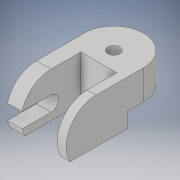
# Autodesk Inventor part: knuckle
Saved by Autodesk Inventor 2018 (Build 220112000, 112)
## iProperties
Created: 2017-10-01
Part Number: knuckle
Material: Generic
Document SubType Name: Modeling
Designer: Martin
Density: 1 g/cm^3
Appearance: Default
Author: Martin
Autodesk Inventor part; units mm, degrees
ref_plane "YZ Plane" through (0, 0, 0) normal (1, 0, 0) x (0, 1, 0)
ref_plane "XZ Plane" through (0, 0, 0) normal (0, 1, 0) x (-1, 0, 0)
ref_plane "XY Plane" through (0, 0, 0) normal (0, 0, 1) x (1, 0, 0)
sketch "Sketch1" plane through (0, 0, 0) normal (1, 0, 0) x (0, 1, 0)
  point P0 (0, 0)
sketch "Sketch2" plane through (0, 0, 0) normal (1, 0, 0) x (0, 1, 0)
  arc A0 (10, 0) -> (-10, 0) centre (0, 0) ccw
  circle A1 centre (0, 0) radius 1.5
  line L0 (10, 0) -> (-10, 0)
  line L1 (-10, 0) -> (-10, -16)
  line L2 (0, -26) -> (10, -26)
  line L3 (10, -26) -> (10, 0)
  line L4 (0, -26) -> (0, -16)
  line L5 (0, -16) -> (-10, -16)
  dimension "d1" = 3
  constraints: 12 end point, 2 centre point, 2 coincident, 2 parallel, 2 point on circle, 1 horizontal, 1 perpendicular
  measures "d1" diameter of A1
extrude "Extrusion1" add sketch "Sketch2" along normal blind 20
sketch "Sketch3" plane through (0, 10, 0) normal (0, 1, 0) x (1, 0, 0)
  line L0 (0, 26) -> (20, 26) projected
  line L1 (0, 16) -> (20, 16) projected
  arc A0 (20, 16) -> (0, 16) centre (10, 16) ccw
  line L2 (21.9475, 16) -> (-2.9161, 16)
  line L3 (-2.9161, 16) -> (-2.9161, 27.442)
  line L4 (-2.9161, 27.442) -> (21.9475, 27.442)
  line L5 (21.9475, 27.442) -> (21.9475, 16)
  point P0 (0, 0)
  constraints: 10 end point, 2 parallel, 2 point on circle, 1 centre point, 1 horizontal, 1 perpendicular, 1 tangent
extrude "Extrusion2" cut sketch "Sketch3" against normal blind 20 contours L2 L3 L4 L5 A0
sketch "Sketch5" plane through (0, 10, 0) normal (0, 1, 0) x (1, 0, 0)
  line L0 (0, -10) -> (20, -10) projected
  line L1 (0, -10) -> (4.9, -10)
  line L2 (4.9, -10) -> (4.9, 10)
  line L3 (4.9, 10) -> (17, 10)
  line L4 (17, 10) -> (17, -10)
  line L5 (17, -10) -> (4.9, -10)
  point P0 (0, 0)
  dimension "d10" = 4.9
  dimension "d11" = 20
  dimension "d12" = 12.1
  constraints: 10 end point, 3 perpendicular, 3 point on line, 1 collinear
  measures "d10" distance of L1.start L1.end
  measures "d11" distance of L1.end L2.end
  measures "d12" distance of L2.end L3.end
extrude "Extrusion3" cut sketch "Sketch5" against normal blind 20
sketch "Sketch6" plane through (0, 0, 0) normal (-1, 0, 0) x (0, 0, 1)
  arc A0 (0, 2.5) -> (0, -2.5) centre (0, 0) ccw
  line L0 (0, 2.5) -> (12.401, 2.5)
  line L1 (12.401, 2.5) -> (12.401, -2.5)
  line L2 (12.401, -2.5) -> (0, -2.5)
  dimension "d15" = 5
  constraints: 6 end point, 2 point on circle, 1 centre point, 1 coincident, 1 horizontal, 1 parallel, 1 perpendicular
  measures "d15" diameter of A0
extrude "Extrusion4" cut sketch "Sketch6" against normal blind 5
sketch "Sketch7" plane through (0, 0, 0) normal (-1, 0, 0) x (0, 0, 1)
  line L0 (-16, -10) -> (12.5782, -10)
  line L1 (12.5782, -10) -> (12.5782, -5)
  line L2 (12.5782, -5) -> (-16, -5)
  line L3 (-16, -5) -> (-16, -10)
  point P0 (0, 0)
  dimension "d18" = 5
  constraints: 8 end point, 2 parallel, 1 horizontal, 1 perpendicular
  measures "d18" distance of L1.end L0.end
extrude "Extrusion5" cut sketch "Sketch7" against normal through all
sketch "Sketch8" plane through (0, 10, 0) normal (0, 1, 0) x (1, 0, 0)
  line L0 (0, 16) -> (20, 16) projected
  circle A0 centre (10, 16) radius 2
  point P0 (0, 0)
  dimension "d21" = 4
  constraints: 1 centre point, 1 midpoint
  measures "d21" diameter of A0
extrude "Extrusion6" cut sketch "Sketch8" against normal through all
sketch "Sketch9" plane through (0, -5, -16) normal (0, -1, 0) x (1, 0, 0)
  line L0 (0, 0) -> (8, 0) projected
  line L1 (12, 0) -> (20, 0) projected
  line L2 (8, 0) -> (12, 0)
  circle A0 centre (10, 0) radius 4.5
  point P0 (0, 16)
  dimension "d24" = 9
  constraints: 2 end point, 1 centre point, 1 collinear, 1 midpoint
  measures "d24" diameter of A0
extrude "Extrusion7" cut sketch "Sketch9" against normal blind 10
sketch "Sketch12" plane through (0, -5, -16) normal (0, -1, 0) x (1, 0, 0)
  arc A0 (14.5, 0) -> (5.5, 0) centre (10, 0) ccw projected
  line L0 (4.9, 6) -> (17, 6) projected
  line L1 (9, 6) -> (9, 4.2062)
  line L2 (11, 6) -> (11, 4.2062)
  line L3 (9, 4.2062) -> (11, 4.2062)
  line L4 (9, 6) -> (11, 6)
  point P0 (0, 16)
  constraints: 8 end point, 1 collinear, 1 perpendicular
extrude "Extrusion8" cut sketch "Sketch12" against normal blind 4
sketch "Sketch13" plane through (0, -5, -16) normal (0, -1, 0) x (1, 0, 0)
  arc A0 (5.5, 0) -> (-5.5, 0) centre (0, 0) ccw
  arc A1 (25.5, 0) -> (14.5, 0) centre (20, 0) ccw
  line L0 (26.0588, 0) -> (26.0588, -15.4765)
  line L1 (26.0588, -15.4765) -> (-5.5, -15.4765)
  line L2 (-5.5, -15.4765) -> (-5.5, 0)
  line L3 (5.5, 0) -> (14.5, 0)
  line L4 (25.5, 0) -> (26.0588, 0)
  point P0 (0, 16)
  dimension "d33" = 11
  dimension "d34" = 11
  constraints: 10 end point, 4 point on circle, 3 parallel, 2 centre point, 2 horizontal, 2 perpendicular
  measures "d33" diameter of A0
  measures "d34" diameter of A1
extrude "Extrusion9" cut sketch "Sketch13" against normal blind 5
body "Solid1"
